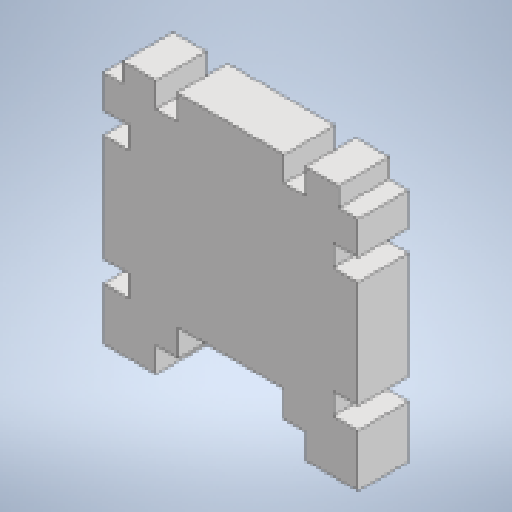
# Autodesk Inventor part: Cemento
Saved by Autodesk Inventor 2024 (Build 280153000, 153)
## iProperties
Created: 2024-07-16
Part Number: Cemento
Material: Genérico
Document SubType Name: Modeling
Designer: sergi
Density: 1 g/cm^3
Appearance: Valor por defecto
Author: sergi
Autodesk Inventor part; units mm, degrees
ref_plane "YZ Plane" through (0, 0, 0) normal (1, 0, 0) x (0, 1, 0)
ref_plane "XZ Plane" through (0, 0, 0) normal (0, 1, 0) x (-1, 0, 0)
sketch "Boceto1" plane through (0, 0, 0) normal (0, 0, 1) x (1, 0, 0)
  line L0 (40.8, -59.2) -> (-40.8, -59.2) projected
  line L1 (40.8, -79.7) -> (40.8, -59.2) projected
  line L2 (99.2, -99.2) -> (58.3, -99.2) projected
  line L3 (99.2, -58.3) -> (99.2, -99.2) projected
  line L4 (58.3, 99.2) -> (99.2, 99.2) projected
  line L5 (-99.2, 58.3) -> (-99.2, 99.2) projected
  line L6 (-58.3, -99.2) -> (-99.2, -99.2) projected
  line L7 (-40.8, -59.2) -> (-40.8, -79.7) projected
  line L8 (-40.8, -79.7) -> (-58.3, -79.7) projected
  line L9 (58.3, -79.7) -> (40.8, -79.7) projected
  line L10 (58.3, -99.2) -> (58.3, -79.7) projected
  line L11 (79.7, -58.3) -> (99.2, -58.3) projected
  line L12 (79.7, -41.7) -> (79.7, -58.3) projected
  line L13 (99.2, -41.7) -> (79.7, -41.7) projected
  line L14 (99.2, 41.7) -> (99.2, -41.7) projected
  line L15 (79.7, 41.7) -> (99.2, 41.7) projected
  line L16 (79.7, 58.3) -> (79.7, 41.7) projected
  line L17 (99.2, 58.3) -> (79.7, 58.3) projected
  line L18 (99.2, 99.2) -> (99.2, 58.3) projected
  line L19 (58.3, 79.7) -> (58.3, 99.2) projected
  line L20 (41.7, 79.7) -> (58.3, 79.7) projected
  line L21 (41.7, 99.2) -> (41.7, 79.7) projected
  line L22 (-41.7, 99.2) -> (41.7, 99.2) projected
  line L23 (-41.7, 79.7) -> (-41.7, 99.2) projected
  line L24 (-58.3, 79.7) -> (-41.7, 79.7) projected
  line L25 (-58.3, 99.2) -> (-58.3, 79.7) projected
  line L26 (-99.2, 99.2) -> (-58.3, 99.2) projected
  line L27 (-79.7, 58.3) -> (-99.2, 58.3) projected
  line L28 (-79.7, 41.7) -> (-79.7, 58.3) projected
  line L29 (-99.2, 41.7) -> (-79.7, 41.7) projected
  line L30 (-99.2, -41.7) -> (-99.2, 41.7) projected
  line L31 (-79.7, -41.7) -> (-99.2, -41.7) projected
  line L32 (-79.7, -58.3) -> (-79.7, -41.7) projected
  line L33 (-99.2, -58.3) -> (-79.7, -58.3) projected
  line L34 (-99.2, -99.2) -> (-99.2, -58.3) projected
  line L35 (-58.3, -79.7) -> (-58.3, -99.2) projected
  line L36 (99.2, 84.2) -> (99.2, 58.3) projected
  line L37 (84.2, 84.2) -> (99.2, 84.2) projected
  line L38 (84.2, 99.2) -> (84.2, 84.2) projected
  line L39 (58.3, 99.2) -> (84.2, 99.2) projected
  line L40 (58.3, 79.7) -> (58.3, 99.2) projected
  line L41 (41.7, 79.7) -> (58.3, 79.7) projected
  line L42 (41.7, 99.2) -> (41.7, 79.7) projected
  line L43 (-41.7, 99.2) -> (41.7, 99.2) projected
  line L44 (-41.7, 79.7) -> (-41.7, 99.2) projected
  line L45 (-58.3, 79.7) -> (-41.7, 79.7) projected
  line L46 (-58.3, 99.2) -> (-58.3, 79.7) projected
  line L47 (-84.2, 99.2) -> (-58.3, 99.2) projected
  line L48 (-84.2, 84.2) -> (-84.2, 99.2) projected
  line L49 (-99.2, 84.2) -> (-84.2, 84.2) projected
  line L50 (-99.2, 58.3) -> (-99.2, 84.2) projected
  line L51 (-79.7, 58.3) -> (-99.2, 58.3) projected
  line L52 (-79.7, 41.7) -> (-79.7, 58.3) projected
  line L53 (-99.2, 41.7) -> (-79.7, 41.7) projected
  line L54 (-99.2, -41.7) -> (-99.2, 41.7) projected
  line L55 (-79.7, -41.7) -> (-99.2, -41.7) projected
  line L56 (-79.7, -58.3) -> (-79.7, -41.7) projected
  line L57 (-99.2, -58.3) -> (-79.7, -58.3) projected
  line L58 (-99.2, -99.2) -> (-99.2, -58.3) projected
  line L59 (-58.3, -99.2) -> (-99.2, -99.2) projected
  line L60 (-58.3, -79.7) -> (-58.3, -99.2) projected
  line L61 (-40.8, -79.7) -> (-58.3, -79.7) projected
  line L62 (-40.8, -59.2) -> (-40.8, -79.7) projected
  line L63 (40.8, -59.2) -> (-40.8, -59.2) projected
  line L64 (40.8, -79.7) -> (40.8, -59.2) projected
  line L65 (58.3, -79.7) -> (40.8, -79.7) projected
  line L66 (58.3, -99.2) -> (58.3, -79.7) projected
  line L67 (99.2, -99.2) -> (58.3, -99.2) projected
  line L68 (99.2, -58.3) -> (99.2, -99.2) projected
  line L69 (79.7, -58.3) -> (99.2, -58.3) projected
  line L70 (79.7, -41.7) -> (79.7, -58.3) projected
  line L71 (99.2, -41.7) -> (79.7, -41.7) projected
  line L72 (99.2, 41.7) -> (99.2, -41.7) projected
  line L73 (79.7, 41.7) -> (99.2, 41.7) projected
  line L74 (79.7, 58.3) -> (79.7, 41.7) projected
  line L75 (99.2, 58.3) -> (79.7, 58.3) projected
  line L76 (-99.2, 58.3) -> (-99.2, 84.2)
  line L77 (99.2, 84.2) -> (99.2, 58.3) projected
  line L78 (84.2, 84.2) -> (99.2, 84.2) projected
  line L79 (84.2, 99.2) -> (84.2, 84.2) projected
  line L80 (58.3, 99.2) -> (84.2, 99.2) projected
  line L81 (58.3, 79.7) -> (58.3, 99.2) projected
  line L82 (41.7, 79.7) -> (58.3, 79.7) projected
  line L83 (41.7, 99.2) -> (41.7, 79.7) projected
  line L84 (-41.7, 99.2) -> (41.7, 99.2) projected
  line L85 (-41.7, 79.7) -> (-41.7, 99.2) projected
  line L86 (-58.3, 79.7) -> (-41.7, 79.7) projected
  line L87 (-58.3, 99.2) -> (-58.3, 79.7) projected
  line L88 (-84.2, 99.2) -> (-58.3, 99.2) projected
  line L89 (-84.2, 84.2) -> (-84.2, 99.2) projected
  line L90 (-99.2, 84.2) -> (-84.2, 84.2) projected
  line L91 (-99.2, 58.3) -> (-99.2, 84.2) projected
  line L92 (-79.7, 58.3) -> (-99.2, 58.3) projected
  line L93 (-79.7, 41.7) -> (-79.7, 58.3) projected
  line L94 (-99.2, 41.7) -> (-79.7, 41.7) projected
  line L95 (-99.2, -41.7) -> (-99.2, 41.7) projected
  line L96 (-79.7, -41.7) -> (-99.2, -41.7) projected
  line L97 (-79.7, -58.3) -> (-79.7, -41.7) projected
  line L98 (-99.2, -58.3) -> (-79.7, -58.3) projected
  line L99 (-99.2, -99.2) -> (-99.2, -58.3) projected
  line L100 (-58.3, -99.2) -> (-99.2, -99.2) projected
  line L101 (-58.3, -79.7) -> (-58.3, -99.2) projected
  line L102 (-40.8, -79.7) -> (-58.3, -79.7) projected
  line L103 (-40.8, -59.2) -> (-40.8, -79.7) projected
  line L104 (40.8, -59.2) -> (-40.8, -59.2) projected
  line L105 (40.8, -79.7) -> (40.8, -59.2) projected
  line L106 (58.3, -79.7) -> (40.8, -79.7) projected
  line L107 (58.3, -99.2) -> (58.3, -79.7) projected
  line L108 (99.2, -99.2) -> (58.3, -99.2) projected
  line L109 (99.2, -58.3) -> (99.2, -99.2) projected
  line L110 (79.7, -58.3) -> (99.2, -58.3) projected
  line L111 (79.7, -41.7) -> (79.7, -58.3) projected
  line L112 (99.2, -41.7) -> (79.7, -41.7) projected
  line L113 (99.2, 41.7) -> (99.2, -41.7) projected
  line L114 (79.7, 41.7) -> (99.2, 41.7) projected
  line L115 (79.7, 58.3) -> (79.7, 41.7) projected
  line L116 (99.2, 58.3) -> (79.7, 58.3) projected
  line L117 (99.2, 84.2) -> (99.2, 58.3) projected
  line L118 (84.2, 84.2) -> (99.2, 84.2) projected
  line L119 (84.2, 99.2) -> (84.2, 84.2) projected
  line L120 (58.3, 99.2) -> (84.2, 99.2) projected
  line L121 (58.3, 79.7) -> (58.3, 99.2) projected
  line L122 (41.7, 79.7) -> (58.3, 79.7) projected
  line L123 (41.7, 99.2) -> (41.7, 79.7) projected
  line L124 (-41.7, 99.2) -> (41.7, 99.2) projected
  line L125 (-41.7, 79.7) -> (-41.7, 99.2) projected
  line L126 (-58.3, 79.7) -> (-41.7, 79.7) projected
  line L127 (-58.3, 99.2) -> (-58.3, 79.7) projected
  line L128 (-84.2, 99.2) -> (-58.3, 99.2) projected
  line L129 (-84.2, 84.2) -> (-84.2, 99.2) projected
  line L130 (-99.2, 84.2) -> (-84.2, 84.2) projected
  line L131 (-99.2, 58.3) -> (-99.2, 84.2) projected
  line L132 (-79.7, 58.3) -> (-99.2, 58.3) projected
  line L133 (-79.7, 41.7) -> (-79.7, 58.3) projected
  line L134 (-99.2, 41.7) -> (-79.7, 41.7) projected
  line L135 (-99.2, -41.7) -> (-99.2, 41.7) projected
  line L136 (-79.7, -41.7) -> (-99.2, -41.7) projected
  line L137 (-79.7, -58.3) -> (-79.7, -41.7) projected
  line L138 (-99.2, -58.3) -> (-79.7, -58.3) projected
  line L139 (-99.2, -99.2) -> (-99.2, -58.3) projected
  line L140 (-58.3, -99.2) -> (-99.2, -99.2) projected
  line L141 (-58.3, -79.7) -> (-58.3, -99.2) projected
  line L142 (-40.8, -79.7) -> (-58.3, -79.7) projected
  line L143 (-40.8, -59.2) -> (-40.8, -79.7) projected
  line L144 (40.8, -59.2) -> (-40.8, -59.2) projected
  line L145 (40.8, -79.7) -> (40.8, -59.2) projected
  line L146 (58.3, -79.7) -> (40.8, -79.7) projected
  line L147 (58.3, -99.2) -> (58.3, -79.7) projected
  line L148 (99.2, -99.2) -> (58.3, -99.2) projected
  line L149 (99.2, -58.3) -> (99.2, -99.2) projected
  line L150 (79.7, -58.3) -> (99.2, -58.3) projected
  line L151 (79.7, -41.7) -> (79.7, -58.3) projected
  line L152 (99.2, -41.7) -> (79.7, -41.7) projected
  line L153 (99.2, 41.7) -> (99.2, -41.7) projected
  line L154 (79.7, 41.7) -> (99.2, 41.7) projected
  line L155 (79.7, 58.3) -> (79.7, 41.7) projected
  line L156 (99.2, 58.3) -> (79.7, 58.3) projected
  point P0 (0, 0)
  constraints: 2 end point, 1 vertical, 2 other
ref_plane "Plano de trabajo1" through (-100, -100, 39.2) normal (0, 0, 1) x (1, 0, 0)
extrude "Extrusión1" add sketch "Boceto1" along normal up to surface (39.2 mm away) contours L0 L7 L8 L35 L6 L34 L33 L32 L31 L30 L29 L28 L27 L5 L49 L48 L26 L25 L24 L23 L22 L21 L20 L19 L4 L38 L37 L18 L17 L16 L15 L14 L13 L12 L11 L3 L2 L10 L9 L1
